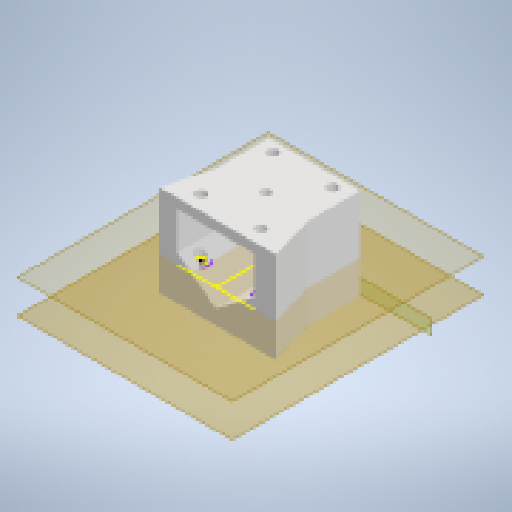
# Autodesk Inventor part: крепеж_маркера
Saved by Autodesk Inventor 2024.2 (Build 282272000, 272)
## iProperties
Created: 2026-01-08
Part Number: крепеж_маркера
Material: Типовые
Document SubType Name: Modeling
Designer: Zakhar
Density: 1 g/cm^3
Appearance: По умолчанию
Author: Zakhar
Autodesk Inventor part; units mm, degrees
ref_plane "РабПлоскость2" through (0, 0, -5) normal (0, 0, -1) x (-1, 0, 0)
sketch "Эскиз1" plane through (0, 0, -5) normal (0, 0, -1) x (-1, 0, 0)
  line L0 (-19.4986, 4.5741) -> (-16.2986, 4.5741) projected
  line L1 (-1.0261, 4.5741) -> (2.1739, 4.5741) projected
  line L2 (-25.5748, 4.5741) -> (-23.7748, 4.5741) projected
  line L3 (5.4196, 4.5741) -> (7.2196, 4.5741) projected
  line L4 (-20.4986, 4.5741) -> (3.1739, 4.5741)
  line L5 (3.1739, 4.5741) -> (3.1739, 9.0001)
  line L6 (3.1739, 9.0001) -> (-20.4986, 9.0001)
  line L7 (-20.4986, 9.0001) -> (-20.4986, 4.5741)
  line L8 (-38.6624, 4.5741) -> (21.3376, 4.5741) projected
  point P0 (0, 0)
  point P1 (-20.4986, 6.7871)
  point P2 (3.1739, 6.7871)
  dimension "d0" = 1
  dimension "d1" = 1
  dimension "d3" = 4.426
  constraints: 8 end point, 2 horizontal, 2 midpoint, 2 parallel, 1 perpendicular, 1 other
  measures "d0" horizontal distance of point (-20.499, 6.787) L0.start
  measures "d1" horizontal distance of point (3.174, 6.787) L1.end
  measures "d3" distance of L4.end L5.end
extrude "Выдавливание1" add sketch "Эскиз1" against normal blind 30
ref_plane "РабПлоскость3" through (5.0978, 4.5741, 0.0339) normal (0, 1, 0) x (-1, 0, 0)
sketch "Эскиз3" plane through (0, 0, 25) normal (0, 0, 1) x (1, 0, 0)
  line L0 (20.4986, 4.5741) -> (20.4986, 9.0001) projected
  line L1 (20.4986, 9.0001) -> (20.4986, 18.0001)
  line L2 (20.4986, 18.0001) -> (8.6624, 9.0001)
  line L3 (20.4986, 9.0001) -> (-3.1739, 9.0001) projected
  line L4 (-3.1739, 9.0001) -> (-3.1739, 4.5741) projected
  line L5 (-3.1739, 18.0001) -> (-3.1739, 9.0001)
  line L6 (-3.1739, 18.0001) -> (8.6624, 9.0001)
  point P0 (0, 0)
  dimension "d8" = 9
  dimension "d9" = 9
  constraints: 8 end point, 1 collinear, 1 midpoint, 1 vertical
  measures "d8" distance of L0.end L1.end
  measures "d9" distance of L5.start L3.end
extrude "Выдавливание3" add sketch "Эскиз3" against normal up to surface (30 mm away)
ref_plane "РабПлоскость4" through (5.0978, 14.8061, 0.0339) normal (0, 1, 0) x (-1, 0, 0)
sketch "Эскиз2" plane through (5.0978, 4.5741, 0.0339) normal (0, 1, 0) x (-1, 0, 0)
  circle A0 centre (-31.4768, 2.1354) radius 0.9
  circle A1 centre (23.5157, 1.4536) radius 0.9
  circle A2 centre (-19.4778, 1.9866) radius 0.9
  circle A3 centre (-19.5769, -6.0128) radius 0.9
  circle A4 centre (23.4165, -6.5458) radius 0.9
  circle A5 centre (11.5166, 1.6023) radius 0.9
  circle A6 centre (11.4174, -6.3971) radius 0.9
  circle A7 centre (-31.576, -5.864) radius 0.9
  circle A8 centre (-12.8008, -1.6339) radius 1.6
  circle A9 centre (5.6717, -1.6339) radius 1.6
  circle A10 centre (-12.8008, 20.3661) radius 1.6
  circle A11 centre (5.6717, 20.3661) radius 1.6
  arc A12 (11.4355, 36.4061) -> (11.4355, 44.3661) centre (11.4355, 40.3861) ccw
  line L0 (11.4355, 44.3661) -> (-18.5645, 44.3661)
  arc A13 (-18.5645, 44.3661) -> (-18.5645, 36.4061) centre (-18.5645, 40.3861) ccw
  line L1 (-18.5645, 36.4061) -> (11.4355, 36.4061)
  line L2 (-33.5645, -20.6339) -> (-33.5645, 49.3661)
  line L3 (-33.5645, 49.3661) -> (26.4355, 49.3661)
  line L4 (26.4355, 49.3661) -> (26.4355, -20.6339)
  line L5 (26.4355, -20.6339) -> (-33.5645, -20.6339)
  point P0 (5.0978, -0.0339)
  constraints: 14 centre point, 12 end point, 4 horizontal, 4 point on circle, 2 vertical, 36 other
extrude "дырки" cut sketch "Эскиз2" along normal through all contours A8 | A9 | A10 | A11
sketch "Эскиз4" plane through (5.0978, 14.8061, 0.0339) normal (0, 1, 0) x (-1, 0, 0)
  circle A0 centre (-12.8008, -1.6339) radius 1.6 projected
  circle A1 centre (-12.8008, 20.3661) radius 1.6 projected
  line L0 (-15.4008, -5.0339) -> (-3.5645, -5.0339) projected
  line L1 (-3.5645, 24.9661) -> (-3.5645, -5.0339) projected
  line L2 (-15.4008, 24.9661) -> (-3.5645, 24.9661) projected
  line L3 (-15.4008, 24.9661) -> (-15.4008, -5.0339) projected
  circle A2 centre (5.6717, -1.6339) radius 1.6 projected
  circle A3 centre (5.6717, 20.3661) radius 1.6 projected
  line L4 (-3.5645, -5.0339) -> (8.2717, -5.0339) projected
  line L5 (8.2717, 24.9661) -> (8.2717, -5.0339) projected
  line L6 (-3.5645, 24.9661) -> (8.2717, 24.9661) projected
  line L7 (-3.5645, 24.9661) -> (-3.5645, -5.0339) projected
  circle A4 centre (-12.8008, 20.3661) radius 2.1992
  circle A5 centre (5.6717, 20.3661) radius 2.3283
  circle A6 centre (-12.8008, -1.6339) radius 2.1992
  circle A7 centre (5.6717, -1.6339) radius 2.3283
  point P0 (5.0978, -0.0339)
  constraints: 4 centre point, 4 coincident
ref_plane "РабПлоскость5" through (5.0978, 4.5741, 0.0339) normal (0, 1, 0) x (-1, 0, 0)
sketch "Эскиз5" plane through (5.0978, 4.5741, 0.0339) normal (0, 1, 0) x (-1, 0, 0)
  line L0 (-15.4008, -5.0339) -> (-3.5645, -5.0339) projected
  line L1 (-3.5645, 24.9661) -> (-3.5645, -5.0339) projected
  line L2 (-15.4008, 24.9661) -> (-3.5645, 24.9661) projected
  line L3 (-15.4008, 24.9661) -> (-15.4008, -5.0339) projected
  line L4 (-3.5645, -5.0339) -> (8.2717, -5.0339) projected
  line L5 (8.2717, 24.9661) -> (8.2717, -5.0339) projected
  line L6 (-3.5645, 24.9661) -> (8.2717, 24.9661) projected
  line L7 (-3.5645, 24.9661) -> (-3.5645, -5.0339) projected
  line L8 (-15.4008, -5.0339) -> (-18, -5.0339)
  line L9 (-18, -5.0339) -> (-18, 24.9661)
  line L10 (-18, 24.9661) -> (-15.4008, 24.9661)
  line L11 (-15.4008, 24.9661) -> (-15.4008, -5.0339)
  line L12 (8.2717, 24.9661) -> (10.1117, 24.9661)
  line L13 (10.1117, 24.9661) -> (10.1117, -5)
  line L14 (10.1117, -5) -> (8.2717, -5)
  line L15 (8.2717, -5) -> (8.2717, 24.9661)
  line L16 (10.1117, 11) -> (13.7176, 11)
  line L17 (13.7176, 11) -> (13.7176, 24.9661)
  line L18 (13.7176, 24.9661) -> (10.1117, 24.9661)
  line L19 (10.1117, 24.9661) -> (10.1117, 11)
  line L20 (-18, 11) -> (-22, 11)
  line L21 (-22, 11) -> (-22, 24.9661)
  line L22 (-22, 24.9661) -> (-18, 24.9661)
  line L23 (-18, 24.9661) -> (-18, 11)
  line L24 (-22, 24.9661) -> (-18, 11)
  line L25 (10.1117, 11) -> (13.7176, 24.9661)
  point P0 (5.0978, -0.0339)
  point P1 (-15.4008, 24.9661)
  point P2 (8.2717, -5)
  dimension "d22" = 1.84
  constraints: 36 end point, 8 parallel, 5 point on line, 4 horizontal, 4 perpendicular
  measures "d22" distance between parallel lines of L13 L15
extrude "Выдавливание5" add sketch "Эскиз5" along normal blind 25 contours L8 L9 L10 L3 | L9 L24 L22 | L12 L13 L14 L5 | L18 L25 L13
sketch "Эскиз6" plane through (5.0978, 29.5741, 0.0339) normal (0, 1, 0) x (1, 0, 0)
  line L0 (15.4008, 5.0339) -> (15.4008, -24.9661) projected
  line L1 (15.4008, -24.9661) -> (22, -24.9661) projected
  line L2 (22, -24.9661) -> (18, -11) projected
  line L3 (18, -11) -> (18, 5.0339) projected
  line L4 (18, 5.0339) -> (15.4008, 5.0339) projected
  line L5 (-13.7176, -24.9661) -> (-8.2717, -24.9661) projected
  line L6 (-8.2717, -24.9661) -> (-8.2717, 5) projected
  line L7 (-8.2717, 5) -> (-10.1117, 5) projected
  line L8 (-10.1117, 5) -> (-10.1117, -11) projected
  line L9 (-10.1117, -11) -> (-13.7176, -24.9661) projected
  line L10 (15.4008, -24.9661) -> (22, -24.9661) projected
  line L11 (15.4008, -24.9661) -> (-8.2717, -24.9661)
  line L12 (18, -11) -> (18, 5.0339) projected
  line L13 (18, 5) -> (-10.1117, 5)
  circle A0 centre (3.8883, -9.9661) radius 1.5
  point P0 (-5.0978, 0.0339)
  dimension "d17" = 15
  dimension "d18" = 14
  dimension "d19" = 3
  constraints: 4 end point, 2 collinear, 2 point on line, 1 centre point, 1 perpendicular
  measures "d17" distance from line of L11 A0.centre
  measures "d18" distance from line of L8 A0.centre
  measures "d19" diameter of A0
extrude "Выдавливание6" add sketch "Эскиз6" along normal blind 3 contours L13 L3 L2 L1 L0 | L0 L11 L6 L13 | L6 L5 L9 L8 L7
sketch "Эскиз7" plane through (5.0978, 32.5741, 0.0339) normal (0, 1, 0) x (1, 0, 0)
  circle A0 centre (12.8008, -20.3661) radius 1.6 projected
  circle A1 centre (-5.6717, -20.3661) radius 1.6 projected
  circle A2 centre (-5.6717, 1.6339) radius 1.6 projected
  circle A3 centre (12.8008, 1.6339) radius 1.6 projected
  point P0 (-5.0978, 0.0339)
extrude "Выдавливание7" cut sketch "Эскиз7" against normal through all
sketch "Эскиз9" plane through (0, 0, -5) normal (0, 0, -1) x (-1, 0, 0)
  line L0 (-23.0978, 4.5741) -> (-23.0978, 29.5741) projected
  line L1 (-23.0978, 29.5741) -> (-20.4986, 29.5741) projected
  line L2 (-20.4986, 29.5741) -> (-20.4986, 18.0001) projected
  line L3 (-20.4986, 18.0001) -> (-8.6624, 9.0001) projected
  line L4 (-8.6624, 9.0001) -> (3.1739, 18.0001) projected
  line L5 (3.1739, 18.0001) -> (3.1739, 4.5741) projected
  line L6 (3.1739, 4.5741) -> (-23.0978, 4.5741) projected
  line L7 (-23.0978, 6.3376) -> (-20.1479, 4.5741)
  line L8 (5.0139, 4.5741) -> (5.0139, 32.5741) projected
  line L9 (5.0139, 6.3376) -> (2.6946, 4.5741)
  line L10 (3.1739, 4.5741) -> (5.0139, 4.5741)
  point P0 (0, 0)
  point P1 (3.1739, 4.9385)
  constraints: 6 end point, 4 point on line, 1 horizontal
extrude "Выдавливание9" cut sketch "Эскиз9" against normal blind 9.25 contours L0 L7 L6 | L5 L9 L8 L10
